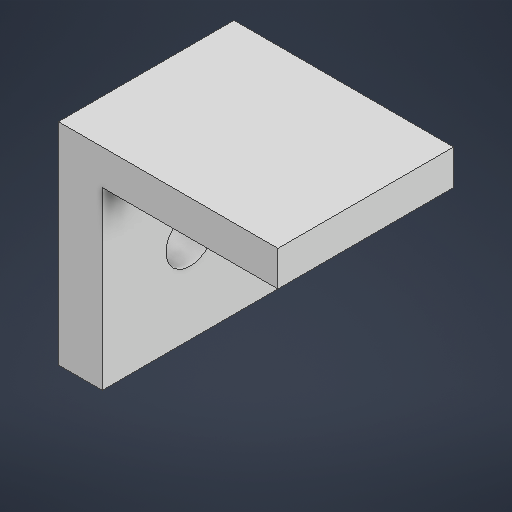
# Autodesk Inventor part: cylinder segment spacer
Saved by Autodesk Inventor 2025 (Build 290162000, 162)
## iProperties
Created: 2024-07-17
Part Number: cylinder segment spacer
Material: Generic
Document SubType Name: Modeling
Designer: mayhe
Density: 1 g/cm^3
Appearance: Default
Author: mayhe
Autodesk Inventor part; units mm, degrees
ref_plane "YZ Plane" through (0, 0, 0) normal (1, 0, 0) x (0, 1, 0)
ref_plane "XZ Plane" through (0, 0, 0) normal (0, 1, 0) x (-1, 0, 0)
ref_plane "XY Plane" through (0, 0, 0) normal (0, 0, 1) x (1, 0, 0)
sketch "Sketch1" plane through (0, 0, 0) normal (0, 0, 1) x (1, 0, 0)
  line L0 (0, 0) -> (0, 24)
  line L1 (0, 24) -> (25, 24)
  line L2 (25, 24) -> (25, 20)
  line L3 (25, 20) -> (5, 20)
  line L4 (5, 20) -> (5, 0)
  line L5 (5, 0) -> (0, 0)
  dimension "d0" = 24
  dimension "d1" = 25
  dimension "d2" = 90
  dimension "d3" = 4
  dimension "d4" = 90
  dimension "d5" = 20
  constraints: 12 end point, 5 perpendicular, 1 vertical
  measures "d0" distance of L0.start L0.end
  measures "d1" distance of L0.end L1.end
  measures "d2" angle of L0 L1
  measures "d3" distance of L1.end L2.end
  measures "d4" angle of L1 L2
  measures "d5" distance of L2.end L3.end
extrude "Extrusion1" add sketch "Sketch1" along normal mid plane 20
sketch "Sketch2" plane through (5, 0, 10) normal (1, 0, 0) x (0, 0, -1)
  circle A0 centre (10, 10) radius 2.75
  point P0 (10, 0)
  dimension "d8" = 5.5
  constraints: 1 centre point
  measures "d8" diameter of A0
extrude "Extrusion2" cut sketch "Sketch2" against normal blind 20
body "Solid1"
